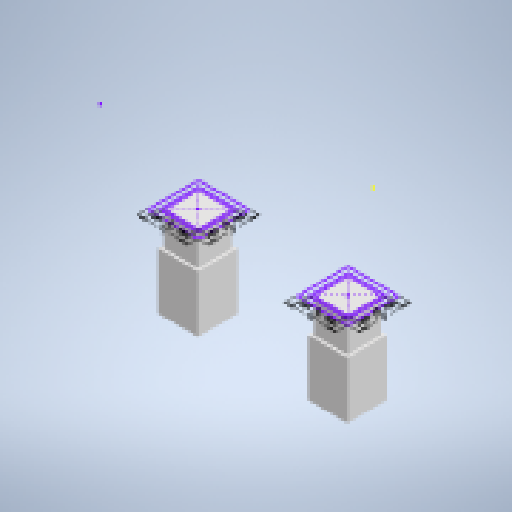
# Autodesk Inventor part: Taster
Saved by Autodesk Inventor 2024 (Build 280153000, 153)
## iProperties
Created: 2025-05-07
Part Number: Taster
Material: Generisch
Document SubType Name: Modeling
Designer: tobia
Density: 1 g/cm^3
Appearance: Vorgabe
Author: tobia
Autodesk Inventor part; units mm, degrees
ref_plane "YZ Plane" through (0, 0, 0) normal (1, 0, 0) x (0, 1, 0)
ref_plane "XZ Plane" through (0, 0, 0) normal (0, 1, 0) x (-1, 0, 0)
ref_plane "XY Plane" through (0, 0, 0) normal (0, 0, 1) x (1, 0, 0)
sketch "Skizze1" plane through (0, 0, 0) normal (0, 0, 1) x (1, 0, 0)
  line L0 (-15.686, -15.3764) -> (-8.686, -15.3764)
  line L1 (-8.686, -15.3764) -> (-8.686, -22.3764)
  line L2 (-8.686, -22.3764) -> (-15.686, -22.3764)
  line L3 (-15.686, -22.3764) -> (-15.686, -15.3764)
  line L4 (-15.686, -15.3764) -> (-8.686, -22.3764) construction
  line L5 (-8.686, -15.3764) -> (-15.686, -22.3764) construction
  line L6 (-16.686, -14.3764) -> (-7.686, -14.3764)
  line L7 (-7.686, -14.3764) -> (-7.686, -23.3764)
  line L8 (-7.686, -23.3764) -> (-16.686, -23.3764)
  line L9 (-16.686, -23.3764) -> (-16.686, -14.3764)
  line L10 (-16.686, -14.3764) -> (-7.686, -23.3764) construction
  line L11 (-7.686, -14.3764) -> (-16.686, -23.3764) construction
  line L12 (-15.186, -15.8764) -> (-9.186, -15.8764)
  line L13 (-9.186, -15.8764) -> (-9.186, -21.8764)
  line L14 (-9.186, -21.8764) -> (-15.186, -21.8764)
  line L15 (-15.186, -21.8764) -> (-15.186, -15.8764)
  line L16 (-15.186, -15.8764) -> (-9.186, -21.8764) construction
  line L17 (-9.186, -15.8764) -> (-15.186, -21.8764) construction
  line L18 (11.2313, -15.8764) -> (17.2313, -15.8764)
  line L19 (17.2313, -15.8764) -> (17.2313, -21.8764)
  line L20 (17.2313, -21.8764) -> (11.2313, -21.8764)
  line L21 (11.2313, -21.8764) -> (11.2313, -15.8764)
  line L22 (11.2313, -15.8764) -> (17.2313, -21.8764) construction
  line L23 (17.2313, -15.8764) -> (11.2313, -21.8764) construction
  line L24 (10.7313, -15.3764) -> (17.7313, -15.3764)
  line L25 (17.7313, -15.3764) -> (17.7313, -22.3764)
  line L26 (17.7313, -22.3764) -> (10.7313, -22.3764)
  line L27 (10.7313, -22.3764) -> (10.7313, -15.3764)
  line L28 (10.7313, -15.3764) -> (17.7313, -22.3764) construction
  line L29 (17.7313, -15.3764) -> (10.7313, -22.3764) construction
  line L30 (9.7313, -14.3764) -> (18.7313, -14.3764)
  line L31 (18.7313, -14.3764) -> (18.7313, -23.3764)
  line L32 (18.7313, -23.3764) -> (9.7313, -23.3764)
  line L33 (9.7313, -23.3764) -> (9.7313, -14.3764)
  line L34 (9.7313, -14.3764) -> (18.7313, -23.3764) construction
  line L35 (18.7313, -14.3764) -> (9.7313, -23.3764) construction
  point P0 (0, 0)
  point P1 (-37.0028, -11.3826)
  point P2 (-12.186, -18.8764)
  point P3 (-12.186, -18.8764)
  point P4 (-12.186, -18.8764)
  point P5 (14.2313, -18.8764)
  point P6 (14.2313, -18.8764)
  point P7 (14.2313, -18.8764)
  dimension "d0" = 7
  dimension "d1" = 7
  dimension "d2" = 9
  dimension "d3" = 9
  dimension "d4" = 6
  dimension "d5" = 6
  dimension "d6" = 6
  dimension "d7" = 6
  dimension "d8" = 7
  dimension "d9" = 7
  dimension "d10" = 9
  dimension "d11" = 9
  constraints: 72 end point, 16 midpoint, 12 parallel, 6 horizontal, 6 perpendicular
  measures "d0" distance of L1.end L2.end
  measures "d1" distance of L0.end L1.end
  measures "d2" distance of L7.end L8.end
  measures "d3" distance of L6.end L7.end
  measures "d4" distance of L13.end L14.end
  measures "d5" distance of L12.end L13.end
  measures "d6" distance of L19.end L20.end
  measures "d7" distance of L18.end L19.end
  measures "d8" distance of L25.end L26.end
  measures "d9" distance of L24.end L25.end
  measures "d10" distance of L31.end L32.end
  measures "d11" distance of L30.end L31.end
extrude "Extrusion1" add sketch "Skizze1" against normal blind 6 contours L12 L13 L14 L15 | L18 L19 L20 L21
sketch "Skizze2" plane through (0, 0, -6) normal (0, 0, -1) x (-1, 0, 0)
  line L0 (9.186, -21.8764) -> (15.186, -21.8764) projected
  line L1 (15.186, -15.8764) -> (9.186, -15.8764) projected
  line L2 (15.186, -21.8764) -> (9.186, -21.8764)
  line L3 (9.186, -21.8764) -> (9.186, -15.8764)
  line L4 (9.186, -15.8764) -> (15.186, -15.8764)
  line L5 (15.186, -15.8764) -> (15.186, -21.8764)
  line L6 (-11.2313, -21.8764) -> (-17.2313, -21.8764) projected
  line L7 (-17.2313, -21.8764) -> (-11.2313, -21.8764)
  line L8 (-11.2313, -21.8764) -> (-11.2313, -15.8764)
  line L9 (-11.2313, -15.8764) -> (-17.2313, -15.8764)
  line L10 (-17.2313, -15.8764) -> (-17.2313, -21.8764)
  line L11 (15.186, -15.8764) -> (12.186, -15.8764)
  line L12 (12.186, -15.8764) -> (12.186, -18.8764)
  line L13 (-11.2313, -15.8764) -> (-14.2313, -15.8764)
  line L14 (-14.2313, -15.8764) -> (-14.2313, -18.8764)
  line L15 (15.686, -22.3764) -> (8.686, -22.3764)
  line L16 (8.686, -22.3764) -> (8.686, -15.3764)
  line L17 (8.686, -15.3764) -> (15.686, -15.3764)
  line L18 (15.686, -15.3764) -> (15.686, -22.3764)
  line L19 (15.686, -22.3764) -> (8.686, -15.3764) construction
  line L20 (8.686, -22.3764) -> (15.686, -15.3764) construction
  line L21 (-10.7313, -22.3764) -> (-17.7313, -22.3764)
  line L22 (-17.7313, -22.3764) -> (-17.7313, -15.3764)
  line L23 (-17.7313, -15.3764) -> (-10.7313, -15.3764)
  line L24 (-10.7313, -15.3764) -> (-10.7313, -22.3764)
  line L25 (-10.7313, -22.3764) -> (-17.7313, -15.3764) construction
  line L26 (-17.7313, -22.3764) -> (-10.7313, -15.3764) construction
  point P0 (0, 0)
  dimension "d15" = 3
  dimension "d16" = 3
  dimension "d17" = 3
  dimension "d18" = 7
  dimension "d19" = 7
  dimension "d20" = 7
  dimension "d21" = 7
  constraints: 48 end point, 8 parallel, 6 midpoint, 6 perpendicular, 4 horizontal
  measures "d15" distance of L4.end L11.end
  measures "d16" distance of L8.end L13.end
  measures "d17" distance of L13.end L14.end
  measures "d18" distance of L16.end L17.end
  measures "d19" distance of L15.end L16.end
  measures "d20" distance of L22.end L23.end
  measures "d21" distance of L21.end L22.end
extrude "Extrusion2" add sketch "Skizze2" along normal blind 9.5 contours L3 L1 L5 L0 | L6 L10 L9 L8 | L15 L16 L17 L18 | L21 L22 L23 L24
